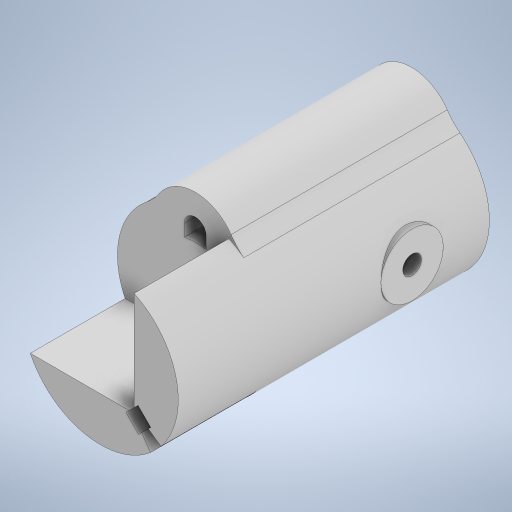
# Autodesk Inventor part: LandingFoot1
Saved by Autodesk Inventor 2023 (Build 270158000, 158)
## iProperties
Created: 2023-01-25
Part Number: LandingFoot1
Material: Generic
Document SubType Name: Modeling
Designer: chase
Density: 1 g/cm^3
Appearance: Default
Author: chase
Autodesk Inventor part; units mm, degrees
ref_plane "YZ Plane" through (0, 0, 0) normal (1, 0, 0) x (0, 1, 0)
sketch "Sketch1" plane through (0, 0, 0) normal (0, 0, 1) x (1, 0, 0)
  circle A0 centre (0, 0) radius 12.5
  dimension "d0" = 25
  constraints: 1 centre point
  measures "d0" diameter of A0
extrude "Extrusion1" add sketch "Sketch1" against normal blind 50
sketch "Sketch2" plane through (0, 0, 0) normal (0, 0, 1) x (1, 0, 0)
  circle A0 centre (0, 0) radius 12.5 projected
  line L0 (0, 12.5) -> (0, 0) construction
  line L1 (0, 0) -> (8.8388, -8.8388) construction
  line L2 (4.5608, -2.5102) -> (9.8641, -7.8135)
  line L3 (9.8641, -7.8135) -> (7.9196, -9.7581)
  line L4 (4.5608, -2.5102) -> (2.5113, -4.5619)
  line L5 (9.8641, -7.8135) -> (7.9196, -9.7581)
  line L6 (8.0964, -6.0458) -> (6.1518, -7.9903)
  line L7 (6.0458, -3.9952) -> (4.1012, -5.9397)
  line L8 (5.4094, -4.6315) -> (3.9244, -3.1466)
  line L9 (4.9497, -4.9497) -> (3.5355, -3.5355)
  line L10 (4.6315, -5.4094) -> (3.1466, -3.9244)
  line L11 (9.4752, -8.2024) -> (7.7075, -6.4347)
  line L12 (8.4146, -9.2631) -> (6.6468, -7.4953)
  line L13 (4.6315, -5.4094) -> (-11.2689, -5.4094)
  line L14 (5.4094, -4.6315) -> (5.4094, 11.2689)
  line L15 (3.3588, -5.4094) -> (2.5113, -4.5619)
  line L16 (7.9196, -9.7581) -> (7.8717, -9.7101)
  line L17 (6.1518, -7.9903) -> (4.1012, -5.9397)
  line L18 (7.7075, -6.4347) -> (9.7869, -7.8907)
  line L19 (6.6468, -7.4953) -> (8.1029, -9.5748)
  point P0 (3.1474, -3.9252)
  point P1 (9.4752, -8.2024)
  point P2 (7.955, -6.1872)
  point P3 (6.1872, -4.4194)
  point P4 (3.9248, -3.147)
  point P5 (5.4094, -3.3588)
  point P6 (9.8045, -7.7539)
  point P7 (8.8388, -8.8388)
  point P8 (8.4044, -9.2529)
  point P9 (9.4523, -8.1795)
  point P10 (9.7281, -7.8495)
  point P11 (8.0779, -9.5392)
  dimension "d12" = 135
  dimension "d14" = 7.5
  dimension "d16" = 7.5
  dimension "d18" = 2.5
  dimension "d19" = 2.9
  dimension "d27" = 1.5
  dimension "d57" = 1.1
  dimension "d58" = 0.55
  dimension "d59" = 1.45
  dimension "d66" = 2.9
  dimension "d68" = 10
  dimension "d69" = 10
  constraints: 40 end point, 11 point on line, 5 perpendicular, 5 point on circle, 4 parallel, 2 collinear, 1 horizontal, 1 tangent, 1 vertical
  measures "d12" angle of L1 L0
  measures "d14" distance of L2.start L2.end
  measures "d16" distance of L3.end L4.end
  measures "d18" distance between parallel lines of L3 L6
  measures "d19" distance between parallel lines of L6 L7
  measures "d27" distance between parallel lines of L12 L11
  measures "d57" distance between parallel lines of L8 L10
  measures "d58" distance between parallel lines of L8 L1
  measures "d59" distance between parallel lines of L9 L2
  measures "d66" distance between parallel lines of L2 L15
  measures "d68" angle of L18 L11
  measures "d69" angle of L12 L19
sketch "Sketch3" plane through (0, 0, -50) normal (0, 0, -1) x (-1, 0, 0)
  circle A0 centre (0, 0) radius 8.075
  circle A1 centre (0, 9.825) radius 1.75
  line L0 (-1.7262, 9.5373) -> (-1.7262, 7.8883)
  line L1 (1.75, 9.8226) -> (1.75, 7.8831)
  dimension "d30" = 16.15
  dimension "d33" = 3.5
  dimension "d65" = 0
  constraints: 4 end point, 4 point on circle, 2 centre point, 1 coincident, 1 parallel, 1 tangent, 1 vertical
  measures "d30" diameter of A0
  measures "d33" diameter of A1
  measures "d65" horizontal distance of point (0, 0) A1.centre
extrude "Extrusion3" cut sketch "Sketch3" against normal blind 25.4 contours A0
extrude "Extrusion4" cut sketch "Sketch3" against normal through all contours A0 A1 L1 | L0 A1 A0 | A1
sketch "Sketch4" plane through (0, 0, -50) normal (0, 0, -1) x (-1, 0, 0)
  arc A0 (6.4405, 10.7131) -> (-6.4161, 10.7277) centre (0.0092, 8.075) ccw
  arc A1 (1.75, 7.8831) -> (-1.7262, 7.8883) centre (0, 0) ccw projected
  circle A2 centre (0, 0) radius 12.5 projected
  point P0 (0.0122, 8.075)
  dimension "d37" = 12.8567
  dimension "d38" = 6.4283
  constraints: 6 point on circle, 1 centre point
  measures "d37" distance of A0.start A0.end
  measures "d38" horizontal distance of A0.start point (0.012, 8.075)
ref_plane "Work Plane1" through (12.5, 0, 0) normal (-1, 0, 0) x (0, 0, 1)
sketch "Sketch6" plane through (12.5, 0, 0) normal (-1, 0, 0) x (0, 0, 1)
  circle A0 centre (-37.5833, 0) radius 5
  point P0 (0, 0)
  dimension "d48" = 10
  constraints: 1 centre point
  measures "d48" diameter of A0
ref_plane "Work Plane2" through (-12.5, 0, 0) normal (1, 0, 0) x (0, 0, -1)
extrude "Extrusion7" add sketch "Sketch6" along normal up to surface (25 mm away)
sketch "Sketch7" plane through (12.5, 0, 0) normal (1, 0, 0) x (0, 0, -1)
  arc A0 (32.5833, 0) -> (42.5833, 0) centre (37.5833, 0) ccw projected
  circle A1 centre (37.5833, 0) radius 1.5
  point P0 (0, 0)
  dimension "d51" = 3
  constraints: 1 centre point, 1 coincident
  measures "d51" diameter of A1
extrude "Extrusion8" cut sketch "Sketch7" against normal through all
sketch "Sketch8" plane through (0, 0, -50) normal (0, 0, -1) x (-1, 0, 0)
  circle A0 centre (0, 0) radius 8.075
  constraints: 1 centre point, 1 coincident
extrude "Extrusion9" cut sketch "Sketch8" against normal up to surface (25.4 mm away)
extrude "Extrusion10" cut sketch "Sketch2" against normal blind 15.24 contours L14 L2 L4 L15 L13 A0 | L14 L8 L4 L2 | A0 L11 L18 | L6 L17 L7 L2 | L15 L4 L10 L13 | L7 L10 L4 L8 | A0 L12 L6 L11 | L19 L12 A0
extrude "Extrusion11" add sketch "Sketch4" against normal up to surface (34.76 mm away) contours A2 A0
fillet "Fillet2" radius 10 2 edges at (6.4161, 10.7277, -32.62) (-6.4405, 10.7131, -32.62)
equation "\"d58\" = 0.5 * d57"
equation "\"d59\" = 0.5 * d66"
equation "\"d38\" = 0.5 * d37"
body "Solid1"
